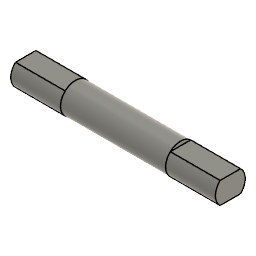
Gearmotor (Autodesk Fusion 360 archive; units mm, degrees)
design "Piece4"
part number: 2026-01-03-02-12-30-808
Autodesk Fusion 360 part; units mm, degrees
note: some values were not read from the file. Chosen so that the rebuilt part matches the saved one: a direction.
sketch "Center" plane through (0, 0, 0) normal (1, 0, 0) x (0, 1, 0)
  circle A0 centre (0, 0) radius 2.7
  dimension "d1" = 5.4
  constraint coincident A0.centre origin
  measures "d1" diameter of A0
extrude "Center width" add sketch "Center" along normal blind 19 makes body 1
sketch "Axis" plane through (19, 0, 0) normal (1, 0, 0) x (0, 1, 0)
  circle A0 centre (0, 0) radius 2.7
  line L0 (-1.85, 1.9666) -> (1.85, 1.9666)
  line L1 (1.85, -1.9666) -> (-1.85, -1.9666)
  arc A1 (-1.85, 1.9666) -> (-1.85, -1.9666) centre (0, 0) ccw
  arc A2 (1.85, -1.9666) -> (1.85, 1.9666) centre (0, 0) ccw
  dimension "d4" = 5.4
  dimension "d5" = 3.7
  constraint coincident A0.centre A1.centre
  constraint horizontal L0
  constraint parallel L0 L1
  constraint coincident A0 L0.start
  constraint concentric A1 A2
  measures "d4" diameter of A1
  measures "d5" distance of L0.start L0.end
extrude "Axis width" add sketch "Axis" along normal blind 9 separate body contours A0 L0 L1 A1 A2 makes body 2
ref_plane "WorkPlane1" through (9.5, 0, 0) normal (1, 0, 0) x (0, 1, 0)
mirror "Axis mirror" about plane through (9.5, 0, 0) normal (1, 0, 0) of "Axis width" makes body 3
equation "d8 = ( 19 / 2 ) * 1 mm"
named bodies: "Center", "Axis part 1", "Axis part 2"

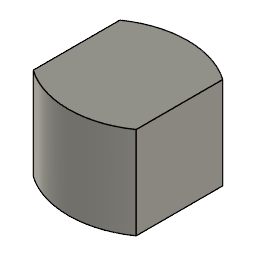
design "Piece5"
part number: 2026-01-03-02-27-47-343
Autodesk Fusion 360 part; units mm, degrees
sketch "Motor base" plane through (0, 0, 0) normal (0, 0, 1) x (1, 0, 0)
  line L0 (0, 0) -> (0, -16)
  line L1 (0, -8) -> (-19, -8) construction
  line L2 (-9.5, -8) -> (-9.5, -19) construction
  line L3 (-19, 0) -> (-19, -16)
  arc A0 (-19, -16) -> (0, -16) centre (-9.5, -2.4583) ccw
  arc A1 (0, 0) -> (-19, 0) centre (-9.5, -13.5417) ccw
  dimension "d1" = 16
  dimension "d2" = 19
  dimension "d3" = 11
  constraint coincident L0.start A1.start
  constraint vertical L0
  constraint midpoint L0 L1.start
  constraint perpendicular L0 L1
  constraint midpoint L1 L2.start
  constraint perpendicular L1 L2
  constraint symmetric L0.start L2 L3.start
  constraint symmetric L0.end L2 L3.end
  constraint coincident L2.end A0
  constraint symmetric L0.end L1 L0.start
  constraint symmetric L1 L3.end L3.start
  constraint symmetric L1 A0 A1
  measures "d1" distance of L0.start L0.end
  measures "d2" distance of L1.start L1.end
  measures "d3" distance of L2.start L2.end
extrude "Motor height" add sketch "Motor base" along normal blind 17
equation "d1 = 22 mm - 6 mm"
named bodies: "Motor"

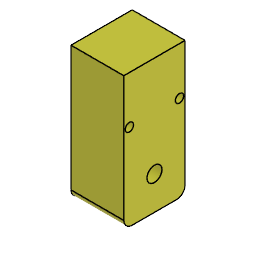
design "Piece3"
part number: 2026-01-03-01-28-17-216
Autodesk Fusion 360 part; units mm, degrees
sketch "Case base" plane through (0, 0, 0) normal (1, 0, 0) x (0, 1, 0)
  line L0 (-11, 24) -> (11, 24)
  line L1 (11, 24) -> (11, -21)
  line L2 (8, -24) -> (-8, -24)
  line L3 (-11, -21) -> (-11, 24)
  line L4 (-11, 24) -> (11, -24) construction
  line L5 (11, 24) -> (-11, -24) construction
  arc A0 (-11, -21) -> (-8, -24) centre (-8, -21) ccw
  arc A1 (8, -24) -> (11, -21) centre (8, -21) ccw
  dimension "d5" = 22
  dimension "d6" = 48
  dimension "d7" = 3
  dimension "d8" = 3
  constraint horizontal L0
  constraint perpendicular L0 L1
  constraint parallel L0 L2
  constraint parallel L1 L3
  constraint coincident L4 origin
  constraint coincident L5 origin
  constraint coincident L5.end L2
  constraint coincident L5.end L3
  constraint tangent L2 A0
  constraint tangent L3 A0
  constraint coincident L4.end L1
  constraint coincident L4.end L2
  constraint tangent L1 A1
  constraint tangent L2 A1
  measures "d5" distance of L4.end L5.end
  measures "d6" distance of L0.start L5.end
  measures "d7" radius of A0
  measures "d8" radius of A1
extrude "Case width" add sketch "Case base" along normal blind 19
sketch "Pin base" plane through (0, 0, -24) normal (0, 0, -1) x (1, 0, 0)
  line L0 (0, 8) -> (0, -8)
  line L1 (0, -8) -> (19, -8)
  line L2 (19, -8) -> (19, 8)
  line L3 (19, 8) -> (0, 8)
  line L4 (0, 0) -> (19, 0) construction
  line L5 (11, 2.5) -> (8, 2.5)
  line L6 (8, 2.5) -> (8, -2.5)
  line L7 (8, -2.5) -> (11, -2.5)
  line L8 (11, -2.5) -> (11, 2.5)
  line L9 (11, 2.5) -> (8, -2.5) construction
  line L10 (8, 2.5) -> (11, -2.5) construction
  point P0 (9.5, 0)
  dimension "d11" = 5
  dimension "d12" = 3
  constraint coincident L4.start origin
  constraint midpoint L2 L4.end
  constraint horizontal L5
  constraint perpendicular L5 L6
  constraint parallel L5 L7
  constraint parallel L6 L8
  constraint coincident L9 P0
  constraint coincident L10 P0
  constraint midpoint L4 P0
  measures "d11" distance of L5.end L6.end
  measures "d12" distance of L5.start L5.end
extrude "Pin base (1)" add sketch "Pin base" along normal blind 5 contours L5 L6 L7 L8
sketch "Pin hole" plane through (11, 0, 0) normal (1, 0, 0) x (0, 1, 0)
  line L0 (2.5, -24) -> (-2.5, -24)
  line L1 (-2.5, -24) -> (-2.5, -29)
  line L2 (-2.5, -29) -> (2.5, -29)
  line L3 (2.5, -29) -> (2.5, -24)
  circle A0 centre (0, -26.5) radius 1.5
  dimension "d15" = 3
  measures "d15" diameter of A0
extrude "Pin hole (1)" cut sketch "Pin hole" against normal through all contours A0
sketch "Case axis" plane through (19, 0, 0) normal (1, 0, 0) x (0, 1, 0)
  arc A0 (-11, -21) -> (-8, -24) centre (-8, -21) ccw
  line L0 (-8, -24) -> (8, -24)
  arc A1 (8, -24) -> (11, -21) centre (8, -21) ccw
  line L1 (11, -21) -> (11, 24)
  line L2 (11, 24) -> (-11, 24)
  line L3 (-11, 24) -> (-11, -21)
  line L4 (0, -24) -> (0, -12) construction
  circle A2 centre (0, -12) radius 2.7
  dimension "d17" = 12
  dimension "d18" = 5.4
  constraint midpoint L0 L4.start
  constraint perpendicular L0 L4
  constraint coincident L4.end A2.centre
  measures "d17" distance of L4.start L4.end
  measures "d18" diameter of A2
extrude "Case axis (1)" cut sketch "Case axis" against normal through all contours A2
sketch "Case hole" plane through (19, 0, 0) normal (1, 0, 0) x (0, 1, 0)
  circle A0 centre (0, -12) radius 2.7
  arc A1 (-11, -21) -> (-8, -24) centre (-8, -21) ccw
  line L0 (-8, -24) -> (8, -24)
  arc A2 (8, -24) -> (11, -21) centre (8, -21) ccw
  line L1 (11, -21) -> (11, 24)
  line L2 (11, 24) -> (-11, 24)
  line L3 (-11, 24) -> (-11, -21)
  line L4 (-11, 22) -> (-9, 22) construction
  line L5 (-9, 24) -> (-9, 7) construction
  circle A3 centre (-9, 7) radius 1.5
  dimension "d20" = 2
  dimension "d21" = 17
  dimension "d22" = 3
  constraint coincident L3 L4.start
  constraint perpendicular L3 L4
  constraint coincident L2 L5.start
  constraint perpendicular L4 L5
  constraint coincident L5.end A3.centre
  measures "d20" distance of L4.start L4.end
  measures "d21" distance of L5.start L5.end
  measures "d22" diameter of A3
extrude "Case hole (1)" cut sketch "Case hole" against normal through all contours A3
mirror "Case holes" about plane through (0, 0, 0) normal (0, 1, 0) of "Case hole (1)"
named bodies: "Case"
